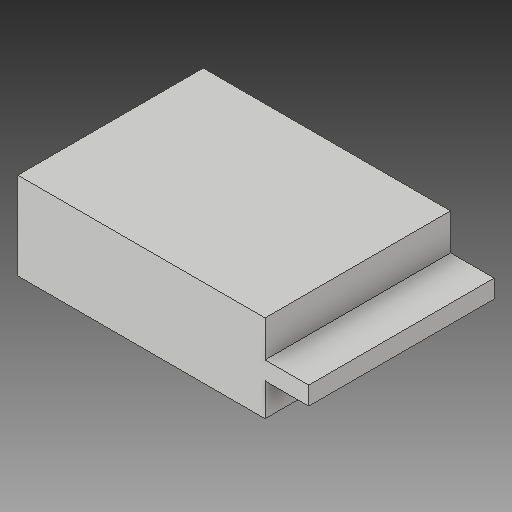
# Autodesk Inventor part: beeper
Saved by Autodesk Inventor 2018 (Build 220112000, 112)
## iProperties
Created: 2017-04-13
Part Number: beeper
Material: Generic
Document SubType Name: Modeling
Designer: steve
Density: 1 g/cm^3
Appearance: Default
Mass: 10.7865 g
Surface Area: 34.98 cm^2
Volume: 10.7865 cm^3
Vendor: HobbyKing
Author: steve
Autodesk Inventor part; units mm, degrees
ref_plane "YZ Plane" through (0, 0, 0) normal (1, 0, 0) x (0, 1, 0)
ref_plane "XZ Plane" through (0, 0, 0) normal (0, 1, 0) x (-1, 0, 0)
ref_plane "XY Plane" through (0, 0, 0) normal (0, 0, 1) x (1, 0, 0)
sketch "Sketch1" plane through (0, 0, 0) normal (0, 1, 0) x (-1, 0, 0)
  line L0 (-17, 12.75) -> (17, 12.75)
  line L1 (17, 12.75) -> (17, -12.75)
  line L2 (17, -12.75) -> (-17, -12.75)
  line L3 (-17, -12.75) -> (-17, 12.75)
  line L4 (-17, 12.75) -> (17, -12.75) construction
  line L5 (17, 12.75) -> (-17, -12.75) construction
  point P0 (0, 0)
  dimension "d0" = 25.5
  dimension "d1" = 34
  constraints: 12 end point, 2 midpoint, 2 parallel, 1 horizontal, 1 perpendicular
  measures "d0" distance of L0.end L1.end
  measures "d1" distance of L1.end L2.end
extrude "Extrusion1" add sketch "Sketch1" along normal blind 12
sketch "Sketch2" plane through (17, 0, 12.75) normal (1, 0, 0) x (0, 0, -1)
  line L0 (0, 0) -> (0, 12) projected
  line L1 (25.5, 0) -> (25.5, 12) projected
  line L2 (0, 7) -> (25.5, 7)
  line L3 (25.5, 7) -> (25.5, 4.5)
  line L4 (25.5, 4.5) -> (0, 4.5)
  line L5 (0, 4.5) -> (0, 7)
  line L6 (0, 12) -> (25.5, 12) projected
  point P0 (12.75, 0)
  dimension "d4" = 2.5
  dimension "d5" = 5
  constraints: 8 end point, 2 parallel, 2 point on line, 1 horizontal, 1 perpendicular
  measures "d4" distance between parallel lines of L2 L4
  measures "d5" distance between parallel lines of L6 L2
extrude "Extrusion2" add sketch "Sketch2" along normal blind 6 contours L0 L2 L1 L4
body "Solid1"
